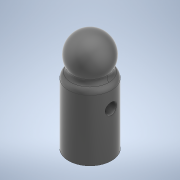
# Autodesk Inventor part: Ballholder
Saved by Autodesk Inventor 2020.2 (Build 242310000, 310)
## iProperties
Created: 2021-06-30
Part Number: Ballholder
Material: Generic
Document SubType Name: Modeling
Designer: JK
Density: 1 g/cm^3
Appearance: Smooth - Black
Author: JK
Autodesk Inventor part; units mm, degrees
ref_plane "YZ Plane" through (0, 0, 0) normal (1, 0, 0) x (0, 1, 0)
ref_plane "XZ Plane" through (0, 0, 0) normal (0, 1, 0) x (-1, 0, 0)
ref_plane "XY Plane" through (0, 0, 0) normal (0, 0, 1) x (1, 0, 0)
sketch "Sketch1" plane through (0, 0, 0) normal (0, 1, 0) x (-1, 0, 0)
  circle A0 centre (0, 0) radius 9.5
  circle A1 centre (0, 0) radius 6.5
  dimension "d0" = 13
  dimension "d1" = 3
  constraints: 2 centre point, 2 coincident
  measures "d0" diameter of A1
  measures "d1" radial gap between concentric circles of A0 A1
extrude "Extrusion1" add sketch "Sketch1" along normal blind 30
sketch "Sketch2" plane through (0, 30, 0) normal (0, 1, 0) x (1, 0, 0)
  circle A0 centre (0, 0) radius 6.5
  constraints: 1 centre point, 1 coincident
extrude "Extrusion2" add sketch "Sketch2" against normal blind 7
sketch "Sketch3" plane through (0, 30, 0) normal (0, 1, 0) x (1, 0, 0)
  circle A0 centre (0, 0) radius 2.2
  dimension "d6" = 4.4
  constraints: 1 centre point, 1 coincident
  measures "d6" diameter of A0
extrude "Extrusion3" [suppressed]
sketch "Sketch6" plane through (0, 0, 0) normal (0, 0, 1) x (1, 0, 0)
  circle A0 centre (0, 36) radius 8.75
  line L0 (6.5, 23) -> (-6.5, 23) projected
  line L1 (9.5, 30) -> (-9.5, 30) projected
  line L2 (0, 0) -> (0, 49.5814)
  point P0 (0, 27.25)
  point P1 (0, 30)
  point P2 (6.3689, 30)
  point P3 (0, 44.75)
  dimension "d24" = 17.5
  dimension "d25" = 6
  dimension "d26" = 0
  constraints: 2 end point, 1 centre point, 1 vertical
  measures "d24" diameter of A0
  measures "d25" distance from line of L1 A0.centre
  measures "d26" horizontal distance of L2.start A0.centre
revolve "Revolution2" add sketch "Sketch6" angle 360 about axis through (0, 0, 0) along (0, 1, 0) picked at (0.649, 39.7602) contours A0 L1 L2
fillet "Fillet5" radius 3 1 edges at (9.5, 30, 0)
fillet "Fillet6" radius 2 1 edges at (-6.3689, 30, 0)
sketch "Sketch8" plane through (0, 23, 0) normal (0, -1, 0) x (1, 0, 0)
  circle A0 centre (0, 0) radius 5.5
  circle A1 centre (0, 0) radius 6.5 projected
  dimension "d34" = 1
  constraints: 1 centre point, 1 coincident
  measures "d34" radial gap between concentric circles of A1 A0
extrude "Extrusion6" add sketch "Sketch8" along normal blind 7
sketch "Sketch7" plane through (0, 0, 0) normal (1, 0, 0) x (0, 1, 0)
  circle A0 centre (20, 0) radius 2.5
  line L0 (27, -9.5) -> (27, 9.5) projected
  point P0 (0, 0)
  dimension "d30" = 5
  dimension "d31" = 7
  constraints: 1 centre point
  measures "d30" diameter of A0
  measures "d31" distance from line of L0 A0.centre
extrude "Extrusion5" cut sketch "Sketch7" along normal blind 10
sketch "Sketch4" plane through (0, 0, 0) normal (1, 0, 0) x (0, 1, 0)
  circle A0 centre (38, 0) radius 8.75
  line L0 (30, -9.5) -> (30, 9.5) projected
  line L1 (12.9825, 0) -> (37.4487, 0)
  point P0 (0, 0)
  point P1 (36.75, 0)
  point P2 (19.25, 0)
  dimension "d9" = 17.5
  dimension "d11" = 8
  constraints: 2 end point, 1 centre point, 1 horizontal
  measures "d9" diameter of A0
  measures "d11" distance from line of A0.centre L0
body "Solid1"
